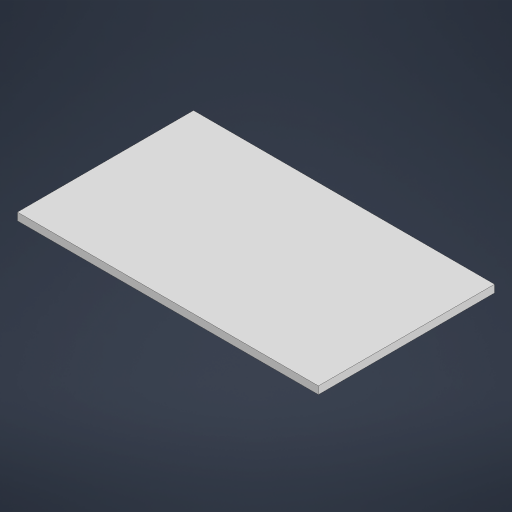
# Autodesk Inventor part: clip-cover
Saved by Autodesk Inventor 2023 (Build 270158000, 158)
## iProperties
Created: 2022-05-18
Part Number: clip-cover
Material: Generic
Document SubType Name: Modeling
Designer: jayso
Density: 1 g/cm^3
Appearance: Default
Author: jayso
Autodesk Inventor part; units mm, degrees
ref_plane "YZ Plane" through (0, 0, 0) normal (1, 0, 0) x (0, 1, 0)
ref_plane "XZ Plane" through (0, 0, 0) normal (0, 1, 0) x (-1, 0, 0)
ref_plane "XY Plane" through (0, 0, 0) normal (0, 0, 1) x (1, 0, 0)
sketch "Sketch2" plane through (0, 0, 0) normal (0, 1, 0) x (-1, 0, 0)
  line L0 (-100, 58.5) -> (-100, -58.5)
  line L1 (-100, -58.5) -> (100, -58.5)
  line L2 (100, -58.5) -> (100, 58.5)
  line L3 (100, 58.5) -> (-100, 58.5)
  point P0 (0, 0)
  point P1 (100, 0)
  dimension "d0" = 117
  dimension "d1" = 200
  dimension "d2" = 58.5
  dimension "d3" = 100
  constraints: 8 end point, 2 parallel, 1 midpoint, 1 perpendicular
  measures "d0" distance of L2.end L1.end
  measures "d1" distance of L1.end L0.end
  measures "d2" distance from line of point (0, 0) L1
  measures "d3" distance of point (0, 0) point (100, 0)
extrude "Extrusion1" add sketch "Sketch2" along normal blind 5
sketch "Sketch3" plane through (0, 0, 0) normal (0, -1, 0) x (1, 0, 0)
  line L0 (94, -52.5) -> (-94, -52.5)
  line L1 (-94, -52.5) -> (-94, 52.5)
  line L2 (-94, 52.5) -> (94, 52.5)
  line L3 (94, 52.5) -> (94, -52.5)
  line L4 (100, -58.5) -> (-100, -58.5) projected
  line L5 (-100, 58.5) -> (100, 58.5) projected
  line L6 (-100, -58.5) -> (-100, 58.5) projected
  line L7 (100, 58.5) -> (100, -58.5) projected
  point P0 (0, 0)
  dimension "d6" = 6
  dimension "d7" = 6
  dimension "d8" = 6
  dimension "d9" = 6
  constraints: 8 end point, 2 parallel, 1 horizontal, 1 perpendicular
  measures "d6" distance between parallel lines of L4 L0
  measures "d7" distance between parallel lines of L5 L2
  measures "d8" distance between parallel lines of L6 L1
  measures "d9" distance between parallel lines of L7 L3
extrude "Extrusion2" add sketch "Sketch3" along normal blind 4 contours L0 L1 L2 L3
fillet "Fillet1" radius 40 4 edges at (94, -2, 52.5) (-94, -2, 52.5) (-94, -2, -52.5) (94, -2, -52.5)
body "Solid1"
